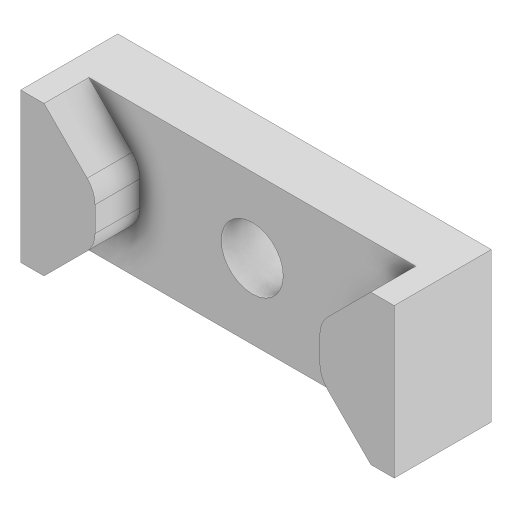
# Autodesk Inventor part: backing_nut
Saved by Autodesk Inventor 2023 (Build 270158000, 158)
## iProperties
Created: 2024-08-28
Part Number: backing_nut
Material: Generic
Document SubType Name: Modeling
Designer: Thomas
Density: 1 g/cm^3
Appearance: Default
Author: Thomas
Autodesk Inventor part; units mm, degrees
ref_plane "YZ Plane" through (0, 0, 0) normal (1, 0, 0) x (0, 1, 0)
ref_plane "XZ Plane" through (0, 0, 0) normal (0, 1, 0) x (-1, 0, 0)
ref_plane "XY Plane" through (0, 0, 0) normal (0, 0, 1) x (1, 0, 0)
sketch "Sketch1" plane through (0, 0, 0) normal (0, 0, 1) x (1, 0, 0)
  circle A0 centre (0, 0) radius 2.075
  line L0 (-12.5, 5) -> (12.5, 5)
  line L1 (12.5, 5) -> (12.5, -5)
  line L2 (12.5, -5) -> (-12.5, -5)
  line L3 (-12.5, -5) -> (-12.5, 5)
  line L4 (-12.5, 5) -> (12.5, -5) construction
  line L5 (12.5, 5) -> (-12.5, -5) construction
  dimension "d0" = 4.15
  dimension "d1" = 25
  dimension "d2" = 10
  constraints: 12 end point, 2 midpoint, 2 parallel, 1 centre point, 1 coincident, 1 horizontal, 1 perpendicular
  measures "d0" diameter of A0
  measures "d1" distance of L1.end L2.end
  measures "d2" distance of L0.end L1.end
extrude "Extrusion1" add sketch "Sketch1" against normal blind 3.5
sketch "Sketch3" plane through (0, 0, 0) normal (0, 0, 1) x (1, 0, 0)
  line L0 (-22.7487, 17.0919) -> (-7.9081, 2.2513)
  arc A0 (-7.3223, 0.837) -> (-7.9081, 2.2513) centre (-9.3223, 0.837) ccw
  line L1 (-7.3223, 0.837) -> (-7.3223, -0.837)
  arc A1 (-7.9081, -2.2513) -> (-7.3223, -0.837) centre (-9.3223, -0.837) ccw
  line L2 (-7.9081, -2.2513) -> (-22.7487, -17.0919)
  line L3 (22.7487, -17.0919) -> (7.9081, -2.2513)
  arc A2 (7.3223, -0.837) -> (7.9081, -2.2513) centre (9.3223, -0.837) ccw
  line L4 (7.3223, -0.837) -> (7.3223, 0.837)
  arc A3 (7.9081, 2.2513) -> (7.3223, 0.837) centre (9.3223, 0.837) ccw
  line L5 (7.9081, 2.2513) -> (22.7487, 17.0919)
  circle A4 centre (0, 0) radius 1.65
  line L6 (-22.7487, 17.0919) -> (-22.7487, -17.0919)
  line L7 (22.7487, 17.0919) -> (22.7487, -17.0919)
  line L8 (-8.0495, 2.1098) -> (-22.5487, 16.609)
  line L9 (-22.5487, 16.609) -> (-22.5487, -16.609)
  line L10 (-22.5487, -16.609) -> (-8.0495, -2.1098)
  arc A5 (-7.5223, 0.837) -> (-8.0495, 2.1098) centre (-9.3223, 0.837) ccw
  line L11 (-7.5223, 0.837) -> (-7.5223, -0.837)
  arc A6 (-8.0495, -2.1098) -> (-7.5223, -0.837) centre (-9.3223, -0.837) ccw
  line L12 (7.5223, -0.837) -> (7.5223, 0.837)
  arc A7 (8.0495, 2.1098) -> (7.5223, 0.837) centre (9.3223, 0.837) ccw
  line L13 (8.0495, 2.1098) -> (22.8902, 16.9505)
  line L14 (22.5487, 17.0919) -> (22.5487, -16.609)
  line L15 (22.5487, -16.609) -> (8.0495, -2.1098)
  arc A8 (7.5223, -0.837) -> (8.0495, -2.1098) centre (9.3223, -0.837) ccw
  line L16 (-12.5, -5) -> (12.5, -5) projected
  line L17 (12.5, -5) -> (12.5, 5) projected
  line L18 (12.5, 5) -> (-12.5, 5) projected
  line L19 (-12.5, 5) -> (-12.5, -5) projected
  circle A9 centre (0, 0) radius 2.075 projected
  point P0 (8.0495, -2.1098)
  point P1 (10.9397, -5)
  point P2 (10.9397, 5)
  point P3 (-10.9397, 5)
  point P4 (-10.9397, -5)
  point P5 (-8.0495, -2.1098)
  dimension "d1" = 25
  dimension "d5" = 0.2
  dimension "d6" = 0.2
  dimension "d7" = 0.2
  dimension "d8" = 0.2
  dimension "d9" = 0.2
  dimension "d10" = 0.2
  dimension "d11" = 0.2
  dimension "d12" = 0.2
  dimension "d13" = 0.2
  constraints: 32 end point, 16 point on circle, 9 centre point, 4 parallel, 1 vertical, 3 other
  measures "d5" distance between parallel lines of L0 L8
  measures "d6" radial gap between concentric circles of A0 A5
  measures "d7" distance between parallel lines of L1 L11
  measures "d8" radial gap between concentric circles of A1 A6
  measures "d9" distance between parallel lines of L4 L12
  measures "d10" radial gap between concentric circles of A3 A7
  measures "d11" distance between parallel lines of L5 L13
  measures "d12" distance between parallel lines of L7 L14
  measures "d13" radial gap between concentric circles of A2 A8
extrude "Extrusion2" add sketch "Sketch3" along normal blind 3 contours L8 A5 L11 A6 L10 L16 L19 L18 | L18 L17 L16 L15 A8 L12 A7 L13
equation "\"d6\" = d5"
equation "\"d7\" = d5"
equation "\"d8\" = d5"
equation "\"d9\" = d5"
equation "\"d10\" = d5"
equation "\"d11\" = d5"
equation "\"d12\" = d5"
equation "\"d13\" = d5"
body "Solid1"
